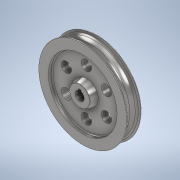
# Autodesk Inventor part: wheel
Saved by Autodesk Inventor 2021 (Build 250183000, 183)
## iProperties
Created: 2022-05-13
Part Number: wheel
Material: Steel, Alloy
Document SubType Name: Modeling
Designer: kajet
Density: 7.73 g/cm^3
Appearance: Semi-Polished
Author: kajet
Autodesk Inventor part; units mm, degrees
ref_plane "YZ Plane" through (0, 0, 0) normal (1, 0, 0) x (0, 1, 0)
ref_plane "XZ Plane" through (0, 0, 0) normal (0, 1, 0) x (-1, 0, 0)
ref_plane "XY Plane" through (0, 0, 0) normal (0, 0, 1) x (1, 0, 0)
sketch "Sketch2" plane through (0, 0, 0) normal (1, 0, 0) x (0, 1, 0)
  arc A0 (175, 25) -> (165, 35) centre (165, 25) ccw
  line L0 (175, 25) -> (176.5, 25)
  line L1 (175, 0) -> (175, 1.25)
  line L2 (175, 1.25) -> (176.5, 1.25)
  line L3 (176.5, 25) -> (176.5, 14.375)
  line L4 (176.5, 14.375) -> (175, 14.375)
  line L5 (175, 14.375) -> (175, 11.875)
  line L6 (175, 11.875) -> (176.5, 11.875)
  line L7 (176.5, 1.25) -> (176.5, 11.875)
  line L8 (176.5, 14.375) -> (176.5, 25)
  line L9 (175, 0) -> (175, 1.25)
  line L10 (175, 11.875) -> (175, 14.375)
  line L11 (165, 35) -> (154.375, 35)
  line L12 (154.375, 35) -> (127.853, 19.6875)
  line L13 (154.375, 35) -> (185, 35) construction
  line L14 (127.853, 19.6875) -> (122.853, 19.6875)
  line L15 (112.5, 0) -> (107.5, 0)
  line L16 (122.853, 19.6875) -> (114.8887, 15.6007)
  arc A1 (110.6738, 11.4897) -> (107.5, 0) centre (133.6725, -1.0464) ccw
  arc A2 (114.8887, 15.6007) -> (110.6738, 11.4897) centre (119.4541, 6.7037) ccw
  line L17 (175, -25) -> (176.5, -25)
  arc A3 (165, -35) -> (175, -25) centre (165, -25) ccw
  line L18 (165, -35) -> (154.375, -35)
  line L19 (154.375, -35) -> (185, -35) construction
  line L20 (176.5, -25) -> (176.5, -14.375)
  line L21 (176.5, -14.375) -> (176.5, -25)
  line L22 (176.5, -14.375) -> (175, -14.375)
  line L23 (175, -14.375) -> (175, -11.875)
  line L24 (175, -11.875) -> (175, -14.375)
  line L25 (175, -11.875) -> (176.5, -11.875)
  line L26 (176.5, -1.25) -> (176.5, -11.875)
  arc A4 (107.5, 0) -> (110.6738, -11.4897) centre (133.6725, 1.0464) ccw
  line L27 (154.375, -35) -> (127.853, -19.6875)
  line L28 (122.853, -19.6875) -> (114.8887, -15.6007)
  arc A5 (110.6738, -11.4897) -> (114.8887, -15.6007) centre (119.4541, -6.7037) ccw
  line L29 (127.853, -19.6875) -> (122.853, -19.6875)
  line L30 (175, 0) -> (175, -1.25)
  line L31 (175, 0) -> (175, -1.25)
  line L32 (175, -1.25) -> (176.5, -1.25)
  line L33 (122.853, 19.6875) -> (92.853, 19.6875)
  line L34 (122.853, 19.6875) -> (92.853, 19.6875)
  line L35 (92.853, 19.6875) -> (92.853, 9.6875)
  line L36 (122.853, -19.6875) -> (92.853, -19.6875)
  line L37 (122.853, -19.6875) -> (92.853, -19.6875)
  line L38 (92.853, -19.6875) -> (92.853, -7.6875)
  line L39 (92.853, 9.6875) -> (32.047, 9.6875)
  line L40 (92.853, -7.6875) -> (32.047, -7.6875)
  line L41 (0, -51.8995) -> (0, 51.8995) projected
  line L42 (57.072, 0) -> (42.072, 0) construction
  line L43 (12.5, 28) -> (12.5, 0)
  line L44 (12.5, 28) -> (27.5033, 28)
  line L45 (32.047, 9.6875) -> (27.5033, 28)
  line L46 (12.5, -28) -> (12.5, 0)
  line L47 (12.5, -28) -> (27.5033, -28)
  line L48 (32.047, -7.6875) -> (27.5033, -28)
  point P0 (0, 0)
  point P1 (0, 0)
  point P2 (175, 35)
  point P3 (112.5, 14.375)
  point P4 (175, -35)
  point P5 (112.5, -14.375)
  dimension "d0" = 35
  dimension "d1" = 10
  dimension "d2" = 1.5
  dimension "d3" = 1.25
  dimension "d4" = 2.5
  dimension "d5" = 10.625
  dimension "d6" = 25
  dimension "d8" = 10.625
  dimension "d9" = 150
  dimension "d10" = 5
  dimension "d11" = 5
  dimension "d12" = 10
  dimension "d16" = 30
  dimension "d17" = 10
  dimension "d42" = 9.6875
  dimension "d43" = 28
  constraints: 96 end point, 16 point on circle, 8 perpendicular, 6 centre point, 6 horizontal, 4 tangent, 3 point on line, 3 vertical, 2 symmetric about line, 1 equal length
  measures "d0" distance of L1.start point (175, 35)
  measures "d1" radius of A0
  measures "d2" distance of L0.start L0.end
  measures "d3" distance of L1.start L1.end
  measures "d4" distance of L4.end L5.end
  measures "d5" distance of L0.end L3.end
  measures "d6" distance of L1.start L0.start
  measures "d8" distance of L11.start L11.end
  measures "d9" angle of L12 L13
  measures "d10" distance of L12.end L14.end
  measures "d11" distance of L15.start L15.end
  measures "d12" radius of A2
  measures "d16" distance of L33.end L14.end
  measures "d17" distance of L33.end L35.end
  measures "d42" distance between parallel lines of L42 L39
  measures "d43" distance of L43.start L43.end
revolve "Revolution4" add sketch "Sketch2" angle 360 about axis through (0, 0, -10) along (0, 0, 1) contours L16 A2 A1 A4 A5 L28 L36 L38 L40 L48 L47 L46 L43 L44 L45 L39 L35 L33
fillet "Fillet3" radius 1 2 edges at (0, -122.853, 19.6875) (0, -122.853, -19.6875)
fillet "Fillet4" radius 1 1 edges at (0, -27.5033, 28)
fillet "Fillet5" radius 3 1 edges at (0, -92.853, 9.6875)
sketch "Sketch7" plane through (0, 0, 28) normal (0, 0, 1) x (1, 0, 0)
  line L0 (0, 20.9459) -> (0, -15.327) construction
  line L1 (-17.5465, 0) -> (23.0283, 0) construction
  circle A0 centre (0, 0) radius 12.5 projected
  line L2 (-4, 9.2) -> (4, 9.2)
  line L3 (4, 9.2) -> (4, 15.8)
  line L4 (4, 15.8) -> (-4, 15.8)
  line L5 (-4, 15.8) -> (-4, 9.2)
  circle A1 centre (0, 0) radius 12.5 projected
  line L6 (-4, 9.2) -> (4, 15.8) construction
  line L7 (4, 9.2) -> (-4, 15.8) construction
  point P0 (0, 12.5)
  point P1 (-4, 11.8427)
  point P2 (4, 11.8427)
  dimension "d44" = 8
  dimension "d45" = 6.6
  constraints: 16 end point, 2 horizontal, 2 midpoint, 2 parallel, 1 perpendicular, 1 vertical, 1 vertical alignment, 1 other
  measures "d44" distance of L4.end L3.end
  measures "d45" distance of L3.end L2.end
extrude "Extrusion3" cut sketch "Sketch7" against normal through all contours A0 L5 L4 L3
sketch "Sketch8" plane through (0, 0, 9.6875) normal (0, 0, 1) x (1, 0, 0)
  line L0 (0, 146.8411) -> (0, -146.8411) construction
  line L1 (-174.8003, 0) -> (222.353, 0) construction
  circle A0 centre (0, 0) radius 62.5 construction
  circle A1 centre (0, 62.5) radius 14
  circle A2 centre (-54.1266, 31.25) radius 14
  circle A3 centre (-54.1266, -31.25) radius 14
  circle A4 centre (0, -62.5) radius 14
  circle A5 centre (54.1266, -31.25) radius 14
  circle A6 centre (54.1266, 31.25) radius 14
  dimension "d48" = 125
  dimension "d49" = 28
  dimension "d52" = 360
  constraints: 6 centre point, 4 end point, 1 coincident, 1 horizontal, 1 point on line, 1 vertical, 1 vertical alignment, 15 other
  measures "d49" diameter of A1
extrude "Extrusion4" cut sketch "Sketch8" against normal through all
body "Solid4"
